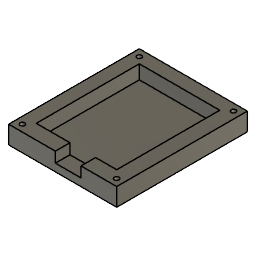
HackYeah (Autodesk Fusion 360 design; units mm, degrees)
part number: 2025-12-04-18-48-26-266
part number: 2025-12-04-19-03-07-969
Autodesk Fusion 360 part; units mm, degrees
sketch "Sketch1" plane through (0, 0, 0) normal (0, 0, 1) x (1, 0, 0) in component "HackYeah (1)"
  line L0 (110, 210) -> (168, 210)
  line L1 (168, 210) -> (168, 135.669)
  line L2 (168, 135.669) -> (110, 135.669)
  line L3 (110, 135.669) -> (110, 210)
  line L4 (100.5, 219.5) -> (178.5, 219.5)
  line L5 (178.5, 219.5) -> (178.5, 125.169)
  line L6 (178.5, 125.169) -> (100.5, 125.169)
  line L7 (100.5, 125.169) -> (100.5, 219.5)
  circle A0 centre (105.5, 130.169) radius 1.7
  circle A1 centre (173.5, 130.169) radius 1.7
  circle A2 centre (105.5, 214.5) radius 1.7
  circle A3 centre (173.5, 214.5) radius 1.7
  circle A4 centre (105.5, 130.169) radius 3
  circle A5 centre (173.5, 130.169) radius 3
  circle A6 centre (105.5, 214.5) radius 3
  circle A7 centre (173.5, 214.5) radius 3
  dimension "d22" = 58
  dimension "d23" = 74.331
  dimension "d24" = 78
  dimension "d25" = 94.331
  dimension "d26" = 9.5
  dimension "d27" = 9.5
  dimension "d28" = 3.4
  dimension "d29" = 5
  dimension "d30" = 5
  dimension "d31" = 3.4
  dimension "d32" = 5
  dimension "d33" = 5
  dimension "d34" = 3.4
  dimension "d35" = 5
  dimension "d36" = 5
  dimension "d37" = 3.4
  dimension "d38" = 5
  dimension "d39" = 5
  dimension "d40" = 6
  dimension "d41" = 6
  dimension "d42" = 6
  dimension "d43" = 6
  constraint horizontal L0
  constraint vertical L1
  constraint horizontal L2
  constraint vertical L3
  constraint horizontal L4
  constraint vertical L5
  constraint horizontal L6
  constraint vertical L7
  constraint concentric A0 A4
  constraint concentric A1 A5
  constraint concentric A2 A6
  constraint concentric A3 A7
  measures "d22" distance of L0.start L0.end
  measures "d23" distance of L0.end L1.end
  measures "d24" distance of L4.start L4.end
  measures "d25" distance of L4.end L5.end
  measures "d26" distance of L0 L4
  measures "d27" distance of L3 L7
  measures "d28" diameter of A0
  measures "d29" distance of L7 A0.centre
  measures "d30" distance of L6 A0.centre
  measures "d31" diameter of A1
  measures "d32" distance of L6 A1.centre
  measures "d33" distance of L5 A1.centre
  measures "d34" diameter of A2
  measures "d35" distance of L4 A2.centre
  measures "d36" distance of L7 A2.centre
  measures "d37" diameter of A3
  measures "d38" distance of L5 A3.centre
  measures "d39" distance of L4 A3.centre
  measures "d40" diameter of A4
  measures "d41" diameter of A5
  measures "d42" diameter of A6
  measures "d43" diameter of A7
extrude "Extrude1" add sketch "Sketch1" along normal blind 9.9 from surface at 3.1 contours A4 | A5 | A6 | A7 makes body 1 at (102.7356, 213.3347, 9.7) makes body 2 at (108.2644, 131.3343, 9.7) makes body 3 at (171.4053, 212.3524, 9.7) makes body 4 at (176.2644, 131.3343, 9.7) in component "HackYeah (1)"
extrude "Extrude2" add sketch "Sketch1" along normal blind 13 contours L4 L5 L6 L7 bodies 1 2 3 4 in component "HackYeah (1)"
extrude "Extrude3" add sketch "Sketch1" along normal blind 3 contours L0 L1 L2 L3 bodies 1 in component "HackYeah (1)"
sketch "Sketch2" plane through (0, 0, 13) normal (0, 0, 1) x (-1, 0, 0) in component "HackYeah (1)"
  circle A0 centre (-105.5, -214.5) radius 1.7
  circle A1 centre (-173.5, -130.169) radius 1.7
  line L0 (-168, -135.669) -> (-110, -135.669)
  line L1 (-110, -135.669) -> (-110, -210)
  line L2 (-110, -210) -> (-168, -210)
  line L3 (-168, -210) -> (-168, -135.669)
  line L4 (-100.5, -125.169) -> (-178.5, -125.169)
  line L5 (-178.5, -125.169) -> (-178.5, -219.5)
  line L6 (-178.5, -219.5) -> (-100.5, -219.5)
  line L7 (-100.5, -219.5) -> (-100.5, -125.169)
  circle A2 centre (-105.5, -130.169) radius 1.7
  circle A3 centre (-173.5, -214.5) radius 1.7
  line L8 (24.854, 25.8508) -> (43.354, 25.8508)
  line L9 (43.354, 25.8508) -> (43.354, 16.3508)
  line L10 (43.354, 16.3508) -> (24.854, 16.3508)
  line L11 (24.854, 16.3508) -> (24.854, 25.8508)
  line L12 (-152.75, -125.169) -> (-134.25, -125.169)
  line L13 (-134.25, -125.169) -> (-134.25, -135.669)
  line L14 (-134.25, -135.669) -> (-152.75, -135.669)
  line L15 (-152.75, -135.669) -> (-152.75, -125.169)
  dimension "d51" = 18.5
  dimension "d52" = 9.5
  dimension "d53" = 18.5
  dimension "d54" = 10.5
  dimension "d55" = 25.75
  constraint horizontal L8
  constraint vertical L9
  constraint horizontal L10
  constraint vertical L11
  constraint horizontal L12
  constraint vertical L13
  constraint horizontal L14
  constraint vertical L15
  constraint coincident L4 L12.start
  measures "d51" distance of L9 L11
  measures "d52" distance of L8 L10
  measures "d53" distance of L12.start L12.end
  measures "d54" distance of L12 L14
  measures "d55" distance of L5 L15
extrude "Extrude4" cut sketch "Sketch2" against normal blind 7.5 contours L0 L4 L12 L13 L14 L15 bodies 1 in component "HackYeah (1)"
component "HackYeah (1)" placed x (1, 0, 0) y (0, 1, 0) z (0, 0, 1) at (0, 0, 0)
